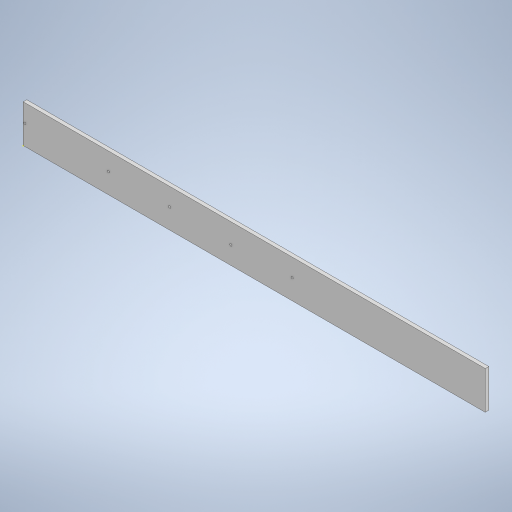
# Autodesk Inventor part: side_support_holder
Saved by Autodesk Inventor 2023 (Build 270158000, 158)
## iProperties
Created: 2022-06-19
Part Number: side_support_holder
Material: Generic
Document SubType Name: Modeling
Designer: prana_p9lsmih
Density: 1 g/cm^3
Appearance: Default
Author: prana_p9lsmih
Autodesk Inventor part; units mm, degrees
ref_plane "YZ Plane" through (0, 0, 0) normal (1, 0, 0) x (0, 1, 0)
ref_plane "XZ Plane" through (0, 0, 0) normal (0, 1, 0) x (-1, 0, 0)
ref_plane "XY Plane" through (0, 0, 0) normal (0, 0, 1) x (1, 0, 0)
sketch "Sketch1" plane through (0, 0, 0) normal (0, 0, 1) x (1, 0, 0)
  line L0 (0, 0) -> (648.5, 0)
  line L1 (648.5, 0) -> (648.5, 53.1557)
  line L2 (648.5, 53.1557) -> (0, 53.1557)
  line L3 (0, 53.1557) -> (0, 0)
  dimension "d21" = 648.5
  constraints: 8 end point, 2 parallel, 1 horizontal, 1 perpendicular
  measures "d21" distance between parallel lines of L1 L3
extrude "Extrusion1" add sketch "Sketch1" along normal blind 5
sketch "Sketch2" plane through (0, 0, 5) normal (0, 0, 1) x (1, 0, 0)
  line L0 (0, 53.1557) -> (0, 0) projected
  line L1 (648.5, 53.1557) -> (0, 53.1557) projected
  line L2 (0, 0) -> (648.5, 0) projected
  point P0 (2.5, 28.1557)
  point P1 (119.44, 28.1557)
  point P2 (205.44, 28.1557)
  point P3 (291.44, 25)
  point P4 (377.44, 28.1557)
  dimension "d4" = 2.5
  dimension "d5" = 25
  dimension "d6" = 119.44
  dimension "d7" = 25
  dimension "d8" = 205.44
  dimension "d9" = 25
  dimension "d10" = 25
  dimension "d11" = 291.44
  dimension "d12" = 25
  dimension "d13" = 377.44
  measures "d4" distance from line of L0 point (2.5, 28.156)
  measures "d5" distance from line of L1 point (2.5, 28.156)
  measures "d6" distance from line of L0 point (119.44, 28.156)
  measures "d7" distance from line of L1 point (119.44, 28.156)
  measures "d8" distance from line of L0 point (205.44, 28.156)
  measures "d9" distance from line of L1 point (205.44, 28.156)
  measures "d10" distance from line of L2 point (291.44, 25)
  measures "d11" distance from line of L0 point (291.44, 25)
  measures "d12" distance from line of L1 point (377.44, 28.156)
  measures "d13" distance from line of L0 point (377.44, 28.156)
hole "Hole1" at (2.5, 28.1557, 5) at (119.44, 28.1557, 5) at (205.44, 28.1557, 5) at (291.44, 25, 5) at (377.44, 28.1557, 5) direction (0, 0, -1) diameter 3 end through all
sketch "Sketch3" plane through (0, 0, 5) normal (0, 0, 1) x (1, 0, 0)
  point P0 (0, 0)
body "Solid1"
